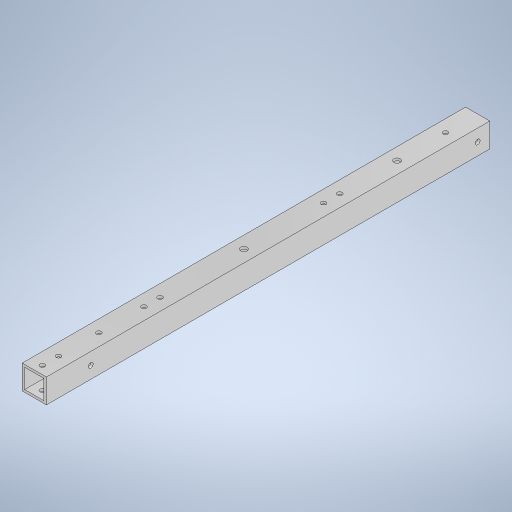
# Autodesk Inventor part: omu_al_jo_6
Saved by Autodesk Inventor 2024.2 (Build 282272000, 272)
## iProperties
Created: 2024-03-23
Part Number: omu_al_jo_6
Material: アルミニウム 6061-AHC
Document SubType Name: Modeling
Designer: fhbdh
Density: 2.7 g/cm^3
Appearance: アルミニウム - ダーク
Author: fhbdh
Autodesk Inventor part; units mm, degrees
ref_plane "YZ Plane" through (0, 0, 0) normal (1, 0, 0) x (0, 1, 0)
ref_plane "XZ Plane" through (0, 0, 0) normal (0, 1, 0) x (-1, 0, 0)
ref_plane "XY Plane" through (0, 0, 0) normal (0, 0, 1) x (1, 0, 0)
derived "omu_sk_jo_1.ipt"
sketch "スケッチ3" plane through (0, 0, 0) normal (0, 1, 0) x (-1, 0, 0)
  circle A0 centre (310.8579, 142.8634) radius 1.5 projected
  line L0 (321.4645, 132.2568) -> (132.2568, 321.4645) construction
  line L1 (243.6827, 321.4645) -> (321.4645, 243.6827) construction
  line L2 (135.7924, 325) -> (325, 135.7924) projected
  line L3 (247.2183, 325) -> (325, 247.2183) projected
  line L4 (317.9289, 128.7213) -> (128.7213, 317.9289) projected
  circle A1 centre (332.5, 257) radius 1.5 projected
  circle A2 centre (332.5, 135.5741) radius 1.5 projected
  circle A3 centre (332.5, 145.5741) radius 1.5 projected
  line L5 (325, 325) -> (325, -325) projected
  line L6 (332.5, 325) -> (332.5, -325) construction
  line L7 (340, -340) -> (340, 340) projected
  line L8 (340, 340) -> (-340, 340) projected
  line L9 (-340, 340) -> (-340, -340) projected
  line L10 (-340, -340) -> (340, 340) construction
  line L11 (340, -340) -> (-340, 340) construction
  line L12 (325, -325) -> (-325, -325) projected
  line L13 (-340, -340) -> (340, -340) projected
  line L14 (325, 135.7924) -> (317.9289, 128.7213) projected
  line L15 (317.9289, 240.1472) -> (325, 247.2183) projected
  circle A4 centre (332.5, 247) radius 1.5 projected
  circle A5 centre (310.8579, 254.2893) radius 1.5 projected
  line L16 (317.9289, 240.1472) -> (240.1472, 317.9289) projected
  circle A6 centre (317.9289, 247.2183) radius 1.5 projected
  line L17 (-325, -325) -> (-325, 325) projected
  line L18 (-325, 325) -> (325, 325) projected
  line L19 (240.1472, 317.9289) -> (247.2183, 325) projected
  line L20 (128.7213, 317.9289) -> (135.7924, 325) projected
  line L21 (325, 332.5) -> (-325, 332.5) construction
  line L22 (262, 310.2183) -> (254.9289, 303.1472) projected
  circle A7 centre (254.2893, 310.8579) radius 1.5 projected
  circle A8 centre (247.2183, 317.9289) radius 1.5 projected
  circle A9 centre (257, 332.5) radius 1.5 projected
  line L23 (262, 340) -> (262, 296.0761) projected
  line L24 (240.1472, 317.9289) -> (240.1472, 340) projected
  circle A10 centre (247, 332.5) radius 1.5 projected
  circle A11 centre (145.5741, 332.5) radius 1.5 projected
  circle A12 centre (142.8634, 310.8579) radius 1.5 projected
  circle A13 centre (135.5741, 332.5) radius 1.5 projected
  circle A14 centre (135.7924, 317.9289) radius 1.5 projected
  circle A15 centre (317.9289, 135.7924) radius 1.5 projected
  line L25 (325, 325) -> (340, 325)
  line L26 (325, 50) -> (340, 50)
  circle A16 centre (332.5, 320) radius 1.5
  circle A17 centre (332.5, 310) radius 1.5
  circle A18 centre (332.5, 285) radius 1.5
  circle A19 centre (332.5, 70) radius 1.5
  point P0 (0, 0)
  point P1 (0, 0)
  dimension "d1" = 275
  dimension "d2" = 3
  dimension "d3" = 10
  dimension "d4" = 5
  dimension "d5" = 3
  dimension "d6" = 40
  dimension "d7" = 3
  dimension "d8" = 255
  constraints: 4 centre point, 4 end point, 3 point on line, 2 perpendicular, 1 equal radius, 5 other
  measures "d1" distance between parallel lines of L25 L26
  measures "d2" diameter of A16
  measures "d3" distance of A17.centre A16.centre
  measures "d4" distance from line of L25 A16.centre
  measures "d5" diameter of A18
  measures "d6" distance from line of L25 A18.centre
  measures "d7" diameter of A19
  measures "d8" distance from line of A19.centre L25
extrude "押し出し2" add sketch "スケッチ3" along normal blind 15 contours L5 L25 L7 L26
sketch "スケッチ4" plane through (-340, 0, 325) normal (0, 0, 1) x (1, 0, 0)
  line L0 (0, 0) -> (15, 0) projected
  line L1 (15, 0) -> (15, 15) projected
  line L2 (0, 15) -> (15, 15) projected
  line L3 (0, 0) -> (0, 15) projected
  line L4 (13.5, 13.5) -> (13.5, 1.5)
  line L5 (13.5, 1.5) -> (1.5, 1.5)
  line L6 (1.5, 1.5) -> (1.5, 13.5)
  line L7 (1.5, 13.5) -> (13.5, 13.5)
  point P0 (340, 0)
  dimension "d13" = 1.5
  constraints: 8 end point, 3 other
  measures "d13" distance between parallel lines of L2 L7
extrude "押し出し3" cut sketch "スケッチ4" against normal through all contours L4 L5 L6 L7
sketch "スケッチ5" plane through (-340, 0, 50) normal (-1, 0, 0) x (0, 0, 1)
  line L0 (0, 0) -> (0, 15) projected
  line L1 (0, 7.5) -> (275, 7.5) construction
  line L2 (275, 0) -> (275, 15) projected
  circle A0 centre (247.5, 7.5) radius 1.5
  circle A1 centre (7.5, 7.5) radius 1.5
  point P0 (-50, 0)
  dimension "d16" = 3
  dimension "d17" = 27.5
  dimension "d18" = 3
  dimension "d19" = 267.5
  constraints: 2 centre point, 2 end point, 2 midpoint, 2 point on line
  measures "d16" diameter of A0
  measures "d17" distance from line of L2 A0.centre
  measures "d18" diameter of A1
  measures "d19" distance from line of L2 A1.centre
extrude "押し出し4" cut sketch "スケッチ5" against normal through all
sketch "スケッチ6" plane through (0, 15, 0) normal (0, 1, 0) x (1, 0, 0)
  line L0 (-340, -325) -> (-325, -325) projected
  line L1 (-332.5, -325) -> (-332.5, -50) construction
  line L2 (-326.5, -50) -> (-338.5, -50) projected
  circle A0 centre (-332.5, -195) radius 2
  circle A1 centre (-332.5, -100) radius 2
  point P0 (0, 0)
  dimension "d22" = 4
  dimension "d23" = 4
  dimension "d24" = 130
  dimension "d25" = 225
  constraints: 3 midpoint, 2 centre point, 2 end point, 2 point on line
  measures "d22" diameter of A0
  measures "d23" diameter of A1
  measures "d24" distance from line of L0 A0.centre
  measures "d25" distance of A1.centre point (-332.5, -325)
extrude "押し出し5" cut sketch "スケッチ6" against normal through all
sketch "スケッチ2" plane through (0, 0, 0) normal (0, 1, 0) x (-1, 0, 0)
  line L0 (-340, -340) -> (340, -340) projected
  line L1 (340, -340) -> (340, 340) projected
  line L2 (340, 340) -> (-340, 340) projected
  line L3 (-340, 340) -> (-340, -340) projected
  line L4 (-340, -340) -> (340, 340) construction
  line L5 (340, -340) -> (-340, 340) construction
  line L6 (325, 325) -> (325, -325) projected
  line L7 (325, -325) -> (-325, -325) projected
  line L8 (-325, -325) -> (-325, 325) projected
  line L9 (-325, 325) -> (325, 325) projected
  line L10 (247.2183, 325) -> (325, 247.2183) projected
  line L11 (317.9289, 240.1472) -> (240.1472, 317.9289) projected
  line L12 (240.1472, 317.9289) -> (247.2183, 325) projected
  line L13 (317.9289, 240.1472) -> (325, 247.2183) projected
  line L14 (135.7924, 325) -> (325, 135.7924) projected
  line L15 (325, 135.7924) -> (317.9289, 128.7213) projected
  line L16 (317.9289, 128.7213) -> (128.7213, 317.9289) projected
  line L17 (128.7213, 317.9289) -> (135.7924, 325) projected
  line L18 (243.6827, 321.4645) -> (321.4645, 243.6827) construction
  line L19 (321.4645, 132.2568) -> (132.2568, 321.4645) construction
  line L20 (325, 332.5) -> (-325, 332.5) construction
  line L21 (332.5, 325) -> (332.5, -325) construction
  circle A0 centre (247.2183, 317.9289) radius 1.5 projected
  circle A1 centre (254.2893, 310.8579) radius 1.5 projected
  circle A2 centre (310.8579, 254.2893) radius 1.5 projected
  circle A3 centre (317.9289, 247.2183) radius 1.5 projected
  circle A4 centre (332.5, 257) radius 1.5 projected
  circle A5 centre (332.5, 247) radius 1.5 projected
  circle A6 centre (257, 332.5) radius 1.5 projected
  circle A7 centre (247, 332.5) radius 1.5 projected
  circle A8 centre (135.7924, 317.9289) radius 1.5 projected
  circle A9 centre (142.8634, 310.8579) radius 1.5 projected
  circle A10 centre (145.5741, 332.5) radius 1.5 projected
  circle A11 centre (135.5741, 332.5) radius 1.5 projected
  circle A12 centre (332.5, 145.5741) radius 1.5 projected
  circle A13 centre (332.5, 135.5741) radius 1.5 projected
  circle A14 centre (317.9289, 135.7924) radius 1.5 projected
  circle A15 centre (310.8579, 142.8634) radius 1.5 projected
  line L22 (240.1472, 317.9289) -> (240.1472, 340) projected
  line L23 (262, 340) -> (262, 296.0761) projected
  line L24 (262, 310.2183) -> (254.9289, 303.1472) projected
  circle A16 centre (332.5, 320) radius 1.5 projected
  circle A17 centre (332.5, 310) radius 1.5 projected
  circle A18 centre (320, 332.5) radius 1.5 projected
  circle A19 centre (310, 332.5) radius 1.5 projected
  point P0 (0, 0)
  point P1 (262, 325)
  point P2 (240.1472, 325)
